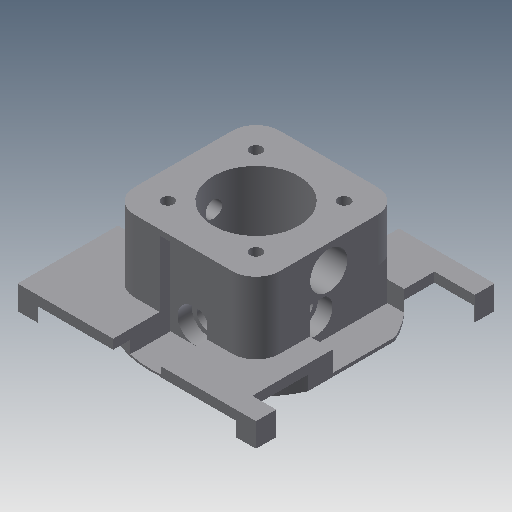
# Autodesk Inventor part: OdourPort_minimal_2_largerhole
Saved by Autodesk Inventor 2018 (Build 220112000, 112)
## iProperties
Created: 2015-07-01
Part Number: OdourPort_minimal_2_largerhole
Material: Generic
Document SubType Name: Modeling
Designer: Janine
Density: 1 g/cm^3
Appearance: Default
Mass: 13.2419 g
Surface Area: 84.1558 cm^2
Volume: 13.2419 cm^3
Author: Janine
Autodesk Inventor part; units mm, degrees
note: some values were not read from the file. Chosen so that the rebuilt part matches the saved one: direction of "Hole10"; direction of "Hole11".
ref_plane "YZ Plane" through (0, 0, 0) normal (1, 0, 0) x (0, 1, 0)
ref_plane "XZ Plane" through (0, 0, 0) normal (0, 1, 0) x (-1, 0, 0)
ref_plane "XY Plane" through (0, 0, 0) normal (0, 0, 1) x (1, 0, 0)
sketch "Sketch1" plane through (0, 0, 0) normal (0, 1, 0) x (-1, 0, 0)
  line L0 (-40, -40) -> (40, -40)
  line L1 (40, -40) -> (40, 40)
  line L2 (40, 40) -> (-40, 40)
  line L3 (-40, 40) -> (-40, -40)
  line L4 (-40, -40) -> (40, 40) construction
  line L5 (40, -40) -> (-40, 40) construction
  line L6 (10, -10) -> (-10, 10) construction
  line L7 (-10, -10) -> (10, 10) construction
  line L8 (15, 15) -> (-15, -15) construction
  line L9 (-15, 15) -> (15, -15) construction
  circle A0 centre (0, 0) radius 15
  dimension "d0" = 80
  dimension "d1" = 80
  dimension "d333" = 30
  constraints: 20 end point, 2 midpoint, 2 parallel, 1 centre point, 1 coincident, 1 horizontal, 1 perpendicular
  measures "d0" distance of L2.end L1.end
  measures "d1" distance of L1.end L0.end
  measures "d333" diameter of A0
extrude "Extrusion1" add sketch "Sketch1" along normal blind 5 contours L3 L2 L1 L0 | A0
sketch "Sketch2" plane through (0, 5, 0) normal (0, 1, 0) x (1, 0, 0)
  line L0 (-20, -20) -> (20, -20)
  line L1 (20, -20) -> (20, 20)
  line L2 (20, 20) -> (-20, 20)
  line L3 (-20, 20) -> (-20, -20)
  line L4 (-20, -20) -> (20, 20) construction
  line L5 (20, -20) -> (-20, 20) construction
  point P0 (0, 0)
  dimension "d330" = 40
  constraints: 12 end point, 2 midpoint
  measures "d330" distance of L0.start L0.end
extrude "Extrusion2" add sketch "Sketch2" along normal blind 15
hole "Hole1" at (0, 0, 0) direction (0, 1, 0) diameter 18 end through all countersink diameter 19 countersink angle 30
hole "Hole10" at (-20, 14, 0) direction (1, 0, 0) diameter 3.5 end up to surface
hole "Hole11" at (20, 15, 0) direction (-1, 0, 0) diameter 7.8 end up to surface
sketch "Sketch11" plane through (20, 5, -20) normal (0, 0, -1) x (-1, 0, 0)
  line L0 (25.0123, -4.5943) -> (25.0123, 13.9057)
  line L1 (25.0123, 13.9057) -> (15.0123, 13.9057)
  line L2 (15.0123, 13.9057) -> (15.0123, -4.5943)
  line L3 (15.0123, -4.5943) -> (25.0123, -4.5943)
  line L4 (0, 15.716) -> (15, 15.716)
  line L5 (20.507, -4.9943) -> (20.507, -4.5943)
  dimension "d173" = 10
  dimension "d174" = 18.5
  dimension "d189" = 15
  dimension "d411" = 0.4
  constraints: 12 end point, 3 perpendicular, 1 point on line, 1 vertical
  measures "d173" distance of L0.end L1.end
  measures "d174" distance of L1.end L2.end
  measures "d189" distance of L4.start L4.end
  measures "d411" distance of L5.start L5.end
extrude "Extrusion11" cut sketch "Sketch11" against normal blind 7
hole "Hole12" at (-0.0123, 3.9, -13) direction (0, 0, 1) diameter 5 depth 10 counterbore diameter 7 counterbore depth 3
sketch "Sketch13" plane through (-12.5061, 5.2672, 20) normal (0, 0, 1) x (1, 0, 0)
  line L0 (17.5572, -4.911) -> (17.5572, 13.589)
  line L1 (17.5572, 13.589) -> (7.5572, 13.589)
  line L2 (7.5572, 13.589) -> (7.5572, -4.911)
  line L3 (7.5572, -4.911) -> (17.5572, -4.911)
  line L4 (-7.4939, 14.7328) -> (7.5061, 14.7328)
  line L5 (-27.4939, -5.2672) -> (52.5061, -5.2672) projected
  line L6 (7.8733, -4.911) -> (7.8733, -5.311)
  dimension "d192" = 10
  dimension "d191" = 18.5
  dimension "d196" = 15
  dimension "d412" = 0.4
  constraints: 12 end point, 4 perpendicular, 1 point on line, 1 vertical
  measures "d192" distance of L0.end L1.end
  measures "d191" distance of L1.end L2.end
  measures "d196" distance of L4.start L4.end
  measures "d412" distance of L6.start L6.end
extrude "Extrusion13" cut sketch "Sketch13" against normal blind 7
hole "Hole14" at (0.0511, 3.9, 13) direction (0, 0, -1) diameter 5 depth 7 counterbore diameter 7 counterbore depth 3
sketch "Sketch14" plane through (-20, 7.482, 14.7328) normal (-1, 0, 0) x (0, 1, 0)
  line L0 (2.5015, 10.7815) -> (2.5015, 29.2815)
  line L1 (2.5015, 29.2815) -> (-7.4985, 29.2815)
  line L2 (-7.4985, 29.2815) -> (-7.4985, 10.7815)
  line L3 (-7.4985, 10.7815) -> (2.5015, 10.7815)
  line L4 (0.0178, 10.7815) -> (0.0178, -5.2672)
  dimension "d208" = 10
  dimension "d207" = 18.5
  constraints: 10 end point
  measures "d208" distance of L0.end L1.end
  measures "d207" distance of L1.end L2.end
extrude "Extrusion14" cut sketch "Sketch14" against normal blind 7
hole "Hole15" at (-13, 4.9835, 0.4513) direction (1, 0, 0) diameter 5 depth 10 counterbore diameter 7 counterbore depth 3
sketch "Sketch15" plane through (20, 14.8049, -20.0315) normal (1, 0, 0) x (0, 1, 0)
  line L0 (-4.1107, 5.4891) -> (-4.1107, 23.9891)
  line L1 (-4.1107, 23.9891) -> (-14.1107, 23.9891)
  line L2 (-14.1107, 23.9891) -> (-14.1107, 5.4891)
  line L3 (-14.1107, 5.4891) -> (-4.1107, 5.4891)
  line L4 (-4.9959, 39.999) -> (-4.9959, 23.999)
  line L5 (-14.8259, 22.2815) -> (-12.8259, 22.2815)
  dimension "d222" = 10
  dimension "d221" = 18.5
  dimension "d410" = 16
  constraints: 12 end point, 3 perpendicular, 1 horizontal
  measures "d222" distance of L0.end L1.end
  measures "d221" distance of L1.end L2.end
  measures "d410" distance of L4.start L4.end
extrude "Extrusion15" cut sketch "Sketch15" against normal blind 7
hole "Hole16" at (13, 5.6942, 0.4576) direction (-1, 0, 0) diameter 5 depth 10 counterbore diameter 7 counterbore depth 3
sketch "Sketch16" plane through (0, 5, 0) normal (0, 1, 0) x (1, 0, 0)
  line L0 (-20, -3.9513) -> (-13, -3.9513) projected
  line L1 (-20, -3.9513) -> (-30, -3.9513)
  line L2 (-30, -3.9513) -> (-30, 14.5487)
  line L3 (-30, 14.5487) -> (-20, 14.5487)
  line L4 (-20, 14.5487) -> (-20, -3.9513)
  point P0 (0, 0)
  dimension "d275" = 10
  dimension "d276" = 18.5
  constraints: 8 end point, 2 parallel, 1 horizontal, 1 perpendicular
  measures "d275" distance of L2.end L3.end
  measures "d276" distance of L1.end L2.end
extrude "Extrusion16" cut sketch "Sketch16" against normal blind 5
sketch "Sketch17" plane through (0, 5, 0) normal (0, 1, 0) x (1, 0, 0)
  line L0 (20, -3.9576) -> (13, -3.9576) projected
  line L1 (20, -3.9576) -> (30, -3.9576)
  line L2 (30, -3.9576) -> (30, 14.5424)
  line L3 (30, 14.5424) -> (20, 14.5424)
  line L4 (20, 14.5424) -> (20, -3.9576)
  point P0 (0, 0)
  dimension "d279" = 10
  dimension "d280" = 18.5
  constraints: 8 end point, 2 parallel, 1 horizontal, 1 perpendicular
  measures "d279" distance of L3.end L2.end
  measures "d280" distance of L2.end L1.end
extrude "Extrusion17" cut sketch "Sketch17" against normal blind 5
sketch "Sketch18" plane through (0, 5, 0) normal (0, 1, 0) x (1, 0, 0)
  line L0 (-20, 20) -> (-5.0123, 20) projected
  line L1 (4.9707, 20) -> (-5.0293, 20)
  line L2 (-5.0293, 20) -> (-5.0293, 30)
  line L3 (-5.0293, 30) -> (4.9707, 30)
  line L4 (4.9707, 30) -> (4.9707, 20)
  point P0 (0, 0)
  point P1 (-15, 20)
  point P2 (15, 20)
  dimension "d302" = 10
  dimension "d303" = 10
  constraints: 8 end point, 2 parallel, 1 horizontal, 1 perpendicular, 1 point on line
  measures "d302" distance of L2.end L3.end
  measures "d303" distance of L1.end L2.end
extrude "Extrusion18" cut sketch "Sketch18" against normal blind 4.6
hole "Hole24" at (-33, 5, -33) direction (0, -1, 0) diameter 5 end through all countersink diameter 9 countersink angle 90
sketch "Sketch19" plane through (0, 5, 0) normal (0, 1, 0) x (1, 0, 0)
  line L0 (5.0511, -20) -> (5.0511, -13) projected
  line L1 (5.0511, -20) -> (-4.9489, -20)
  line L2 (-4.9489, -20) -> (-4.9489, -30)
  line L3 (-4.9489, -30) -> (5.0511, -30)
  line L4 (5.0511, -30) -> (5.0511, -20)
  point P0 (0, 0)
  dimension "d326" = 10
  dimension "d327" = 10
  constraints: 8 end point, 2 parallel, 1 horizontal, 1 perpendicular
  measures "d326" distance of L3.end L2.end
  measures "d327" distance of L2.end L1.end
extrude "Extrusion19" cut sketch "Sketch19" against normal blind 4.6
sketch "Sketch20" plane through (0, 0, 0) normal (0, -1, 0) x (1, 0, 0)
  circle A0 centre (0, 0) radius 22
  circle A1 centre (0, 0) radius 32.5
  dimension "d334" = 44
  dimension "d335" = 65
  constraints: 2 centre point, 2 coincident
  measures "d334" diameter of A0
  measures "d335" diameter of A1
extrude "Extrusion20" cut sketch "Sketch20" against normal blind 3
sketch "Sketch22" plane through (0, 0, 0) normal (0, -1, 0) x (1, 0, 0)
  line L0 (40, 40) -> (40, -40) projected
  line L1 (30, -14.5424) -> (40, -14.5424)
  line L2 (40, -14.5424) -> (40, 22.5261)
  line L3 (40, 22.5261) -> (30, 22.5261)
  line L4 (30, 12.5) -> (30, -14.5424)
  line L5 (30, 22.5261) -> (27.7429, 22.5261)
  arc A0 (30, -12.5) -> (-30, -12.5) centre (0, 0) ccw projected
  line L6 (27.7429, 15.9429) -> (30, 12.5)
  line L7 (27.7429, 22.5261) -> (27.7429, 15.9429)
  point P0 (23.427, 22.5261)
  constraints: 14 end point, 2 horizontal, 2 parallel, 2 point on circle, 1 perpendicular, 1 point on line, 1 vertical
extrude "Extrusion22" cut sketch "Sketch22" against normal through all
sketch "Sketch23" plane through (0, 20, 0) normal (0, 1, 0) x (1, 0, 0)
  line L0 (-15.25, 15.25) -> (15.25, 15.25)
  line L1 (15.25, 15.25) -> (15.25, -15.25)
  line L2 (15.25, -15.25) -> (-15.25, -15.25)
  line L3 (-15.25, -15.25) -> (-15.25, 15.25)
  line L4 (-15.25, 15.25) -> (15.25, -15.25) construction
  line L5 (15.25, 15.25) -> (-15.25, -15.25) construction
  line L6 (-20, -20) -> (20, -20)
  line L7 (20, -20) -> (20, 20)
  line L8 (20, 20) -> (-20, 20)
  line L9 (-20, 20) -> (-20, -20)
  line L10 (-20, -20) -> (20, 20) construction
  line L11 (20, -20) -> (-20, 20) construction
  point P0 (0, 0)
  dimension "d357" = 30.5
  dimension "d359" = 30.5
  constraints: 24 end point, 4 midpoint, 4 parallel, 2 horizontal, 2 perpendicular
  measures "d357" distance of L1.end L2.end
  measures "d359" distance of L0.end L1.end
extrude "Extrusion23" cut sketch "Sketch23" against normal blind 15
sketch "Sketch24" plane through (0, 5, 0) normal (0, 1, 0) x (1, 0, 0)
  line L0 (-25, -25) -> (25, -25)
  line L1 (25, -25) -> (25, 25)
  line L2 (25, 25) -> (-25, 25)
  line L3 (-25, 25) -> (-25, -25)
  circle A0 centre (0, 0) radius 9.5 projected
  line L4 (-25, -25) -> (25, 25) construction
  line L5 (25, -25) -> (-25, 25) construction
  line L6 (40, 14.5424) -> (40, 40) projected
  line L7 (-40, -40) -> (40, -40)
  line L8 (40, -40) -> (40, 40)
  line L9 (40, 40) -> (-40, 40)
  line L10 (-40, 40) -> (-40, -40)
  line L11 (-40, -40) -> (40, 40) construction
  line L12 (40, -40) -> (-40, 40) construction
  point P0 (0, 0)
  dimension "d362" = 50
  dimension "d363" = 50
  constraints: 24 end point, 4 midpoint, 4 parallel, 2 horizontal, 2 perpendicular
  measures "d362" distance of L2.end L1.end
  measures "d363" distance of L1.end L0.end
extrude "Extrusion24" cut sketch "Sketch24" against normal through all contours L8 L7 L10 L9 L6
fillet "Fillet9" radius 5 1 edges at (15.25, 12.5, 15.25)
fillet "Fillet10" radius 5 1 edges at (15.25, 12.5, -15.25)
fillet "Fillet11" radius 5 1 edges at (-15.25, 12.5, -15.25)
fillet "Fillet12" radius 5 1 edges at (-15.25, 12.5, 15.25)
sketch "Sketch25" plane through (0, 0, 0) normal (0, -1, 0) x (1, 0, 0)
  line L0 (25, 3.9576) -> (25, 20.7666) projected
  line L1 (25, -14.5424) -> (25, 20.7666)
  line L2 (25, 20.7666) -> (20, 20.7666)
  line L3 (25, -20.7666) -> (25, -14.5424) projected
  line L4 (16.5422, -14.5993) -> (16.5422, -20.8623)
  line L5 (16.5422, -20.8623) -> (25, -20.8623)
  line L6 (25, -20.8623) -> (25, -14.5424)
  line L7 (20, 20.7666) -> (25, 20.7666)
  arc A0 (16.5082, -14.5424) -> (20, -9.1652) centre (0, 0) ccw projected
  line L8 (16.5082, -14.5424) -> (16.5422, -14.5424)
  line L9 (16.5422, -20.8623) -> (16.5422, -14.5036)
  line L10 (20, 20.7666) -> (20, 3.1121)
  line L11 (20, 3.9576) -> (20, -9.1652) projected
  constraints: 18 end point, 2 point on line, 1 collinear, 1 horizontal, 1 parallel, 1 point on circle, 1 vertical
extrude "Extrusion25" cut sketch "Sketch25" against normal blind 10 contours L1 L3 L6 L5 L4 L9 A0 L11 L10 L2 L0
hole "Hole26" at (-9.25, 20, -9.25) direction (0, -1, 0) diameter 2.5 depth 5 tip angle 118
hole "Hole27" at (-9.25, 20, 9.25) direction (0, -1, 0) diameter 2.5 depth 5 tip angle 118
hole "Hole28" at (9.25, 20, 9.25) direction (0, -1, 0) diameter 2.5 depth 5 tip angle 118
hole "Hole29" at (9.25, 20, -9.25) direction (0, -1, 0) diameter 2.5 depth 5 tip angle 118
body "Solid1"
